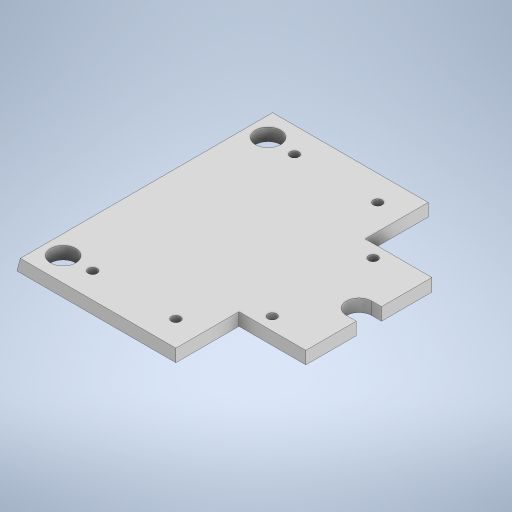
# Autodesk Inventor part: new_plech
Saved by Autodesk Inventor 2024 (Build 280153000, 153)
## iProperties
Created: 2024-01-30
Part Number: new_plech
Material: Všeobecné
Document SubType Name: Modeling
Designer: jaryj
Density: 1 g/cm^3
Appearance: Výchozí
Author: jaryj
Autodesk Inventor part; units mm, degrees
ref_plane "YZ Plane" through (0, 0, 0) normal (1, 0, 0) x (0, 1, 0)
ref_plane "XZ Plane" through (0, 0, 0) normal (0, 1, 0) x (-1, 0, 0)
ref_plane "XY Plane" through (0, 0, 0) normal (0, 0, 1) x (1, 0, 0)
sketch "Náčrt1" plane through (0, 0, 0) normal (0, 1, 0) x (-1, 0, 0)
  line L0 (-50, 50) -> (50, 50)
  line L1 (50, 50) -> (50, -50)
  line L2 (50, -50) -> (-50, -50)
  line L3 (-50, -50) -> (-50, 50)
  line L4 (-50, 50) -> (50, -50) construction
  line L5 (50, 50) -> (-50, -50) construction
  line L6 (-13, 50) -> (-13, 25)
  line L7 (-13, 25) -> (-50, 25)
  line L8 (-50, -25) -> (-13, -25)
  line L9 (-13, -25) -> (-13, -50)
  circle A0 centre (-21.1875, -20) radius 1.75
  circle A1 centre (-21.1875, 20) radius 1.75
  line L10 (-39.5, 25) -> (-39.5, -25)
  circle A2 centre (-3, -40) radius 1.75
  circle A3 centre (30, -40) radius 1.75
  circle A4 centre (30, 40) radius 1.75
  circle A5 centre (-3, 40) radius 1.75
  circle A6 centre (41.083, 40.6105) radius 5
  circle A7 centre (41.083, -40.6105) radius 5
  line L11 (41.083, 40.6105) -> (41.083, 50) construction
  line L12 (41.083, -40.6105) -> (41.083, -50) construction
  circle A8 centre (-35.625, 0) radius 5
  line L13 (-35.625, 5) -> (-39.5, 5)
  line L14 (-35.625, -5) -> (-39.5, -5)
  point P0 (0, 0)
  point P1 (-31.5, 25)
  dimension "d0" = 100
  dimension "d1" = 100
  dimension "d2" = 37
  dimension "d3" = 25
  dimension "d4" = 10.5
  dimension "d5" = 3.5
  dimension "d7" = 10
  dimension "d8" = 10
  dimension "d9" = 5
  dimension "d10" = 5
  dimension "d11" = 10.3125
  dimension "d12" = 10
  dimension "d13" = 20
  dimension "d26" = 81.221
  dimension "d27" = 10
  dimension "d28" = 8.917
  dimension "d29" = 10
  dimension "d30" = 3.875
  constraints: 30 end point, 12 point on line, 9 centre point, 7 perpendicular, 6 equal radius, 4 vertical alignment, 3 horizontal alignment, 3 midpoint, 3 parallel, 2 collinear, 2 point on circle, 2 tangent, 1 horizontal, 1 vertical
  measures "d0" distance of L0.end L1.end
  measures "d1" distance of L1.end L2.end
  measures "d2" distance of L6.end L7.end
  measures "d3" distance of L6.start L6.end
  measures "d4" distance between parallel lines of L10 L3
  measures "d5" diameter of A1
  measures "d7" distance from line of L2 A2.centre
  measures "d8" distance from line of L0 A5.centre
  measures "d9" distance from line of L7 A1.centre
  measures "d10" distance from line of L8 A0.centre
  measures "d11" horizontal distance of A1.centre point (-31.5, 25)
  measures "d12" distance from line of L6 A5.centre
  measures "d13" distance from line of L1 A3.centre
  measures "d26" distance of L12.start L11.start
  measures "d27" diameter of A6
  measures "d28" distance from line of L11.start L1
  measures "d29" diameter of A8
  measures "d30" distance from line of L10 A8.centre
extrude "Vysunutí1" add sketch "Náčrt1" along normal blind 5 contours L0 L1 L2 L9 L8 L10 L14 A8 L13 L7 L6 | A0 | A1 | A2 | A3 | A4 | A5
sketch "Náčrt2" plane through (-50, 0, 50) normal (0, 0, 1) x (1, 0, 0)
  line L0 (0, 0) -> (63, 0) projected
  line L1 (0, 0) -> (1.3397, 5)
  line L2 (0, 5) -> (63, 5) projected
  line L3 (0, 0) -> (0, 5) projected
  line L4 (0, 5) -> (0, 0)
  point P0 (50, 0)
  dimension "d16" = 75
  constraints: 4 end point, 1 point on line, 1 vertical
  measures "d16" angle of L0 L1
extrude "Vysunutí2" cut sketch "Náčrt2" against normal through all
hole "Díra1" at (21.1875, 0, 20) at (21.1875, 0, -20) at (3, 0, -40) at (-30, 0, -40) at (-30, 0, 40) at (3, 0, 40) direction (0, 1, 0) diameter 3.5 end through all countersink diameter 7.5 countersink angle 90
